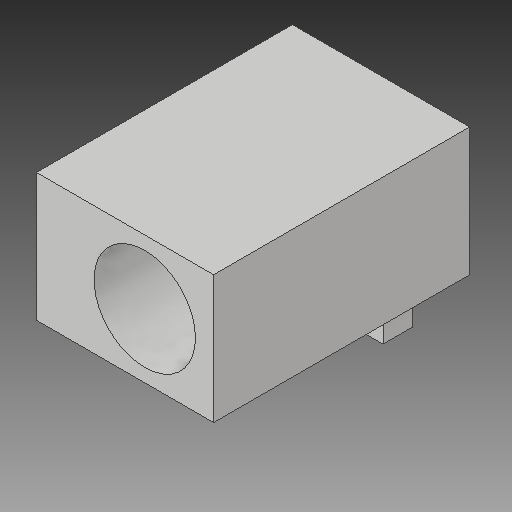
# Autodesk Inventor part: Circuit_DCjack_HEC3110-01-010
Saved by Autodesk Inventor 2018.3 (Build 223284000, 284)
## iProperties
Created: 2018-02-15
Part Number: Circuit_DCjack_HEC3110-01-010
Material: 一般
Document SubType Name: Modeling
Designer: sktom
Density: 1 g/cm^3
Appearance: 既定
Author: sktom
Title: Circuit_DCjack_HEC3110-01-010
Autodesk Inventor part; units mm, degrees
ref_plane "YZ Plane" through (0, 0, 0) normal (1, 0, 0) x (0, 1, 0)
ref_plane "XZ Plane" through (0, 0, 0) normal (0, 1, 0) x (-1, 0, 0)
ref_plane "XY Plane" through (0, 0, 0) normal (0, 0, 1) x (1, 0, 0)
sketch "スケッチ1" plane through (0, 0, 0) normal (0, 0, 1) x (1, 0, 0)
  line L0 (-5.5, 3.25) -> (3.5, 3.25)
  line L1 (3.5, 3.25) -> (3.5, -3.25)
  line L2 (3.5, -3.25) -> (-5.5, -3.25)
  line L3 (-5.5, -3.25) -> (-5.5, 3.25)
  line L4 (-5.5, 3.25) -> (3.5, -3.25) construction
  line L5 (3.5, 3.25) -> (-5.5, -3.25) construction
  circle A0 centre (0, 0) radius 2.575
  point P0 (-1, 0)
  point P1 (-1, 0)
  dimension "d0" = 5.15
  dimension "d1" = 9
  dimension "d2" = 3.5
  dimension "d3" = 6.5
  constraints: 12 end point, 3 midpoint, 2 parallel, 1 centre point, 1 coincident, 1 horizontal, 1 horizontal alignment, 1 perpendicular
  measures "d0" diameter of A0
  measures "d1" distance of L0.start L0.end
  measures "d2" distance from line of point (0, 0) L1
  measures "d3" distance of L0.end L1.end
extrude "押し出し1" add sketch "スケッチ1" against normal blind 13
sketch "スケッチ2" plane through (-5.5, -3.25, 0) normal (0, -1, 0) x (1, 0, 0)
  circle A0 centre (7, -5) radius 0.75
  circle A1 centre (2, -5) radius 0.75
  line L0 (9, 0) -> (0, 0) projected
  point P0 (5.5, 0)
  dimension "d6" = 1.5
  dimension "d7" = 5
  dimension "d8" = 1.5
  dimension "d9" = 3.5
  constraints: 2 centre point, 1 equal radius, 1 horizontal alignment
  measures "d6" diameter of A1
  measures "d7" distance from line of L0 A0.centre
  measures "d8" horizontal distance of point (5.5, 0) A0.centre
  measures "d9" horizontal distance of point (5.5, 0) A1.centre
extrude "押し出し2" add sketch "スケッチ2" along normal blind 1
sketch "スケッチ3" plane through (-5.5, -3.25, 0) normal (0, -1, 0) x (1, 0, 0)
  line L0 (4.15, -10.75) -> (6.85, -10.75)
  line L1 (6.85, -10.75) -> (6.85, -12.25)
  line L2 (6.85, -12.25) -> (4.15, -12.25)
  line L3 (4.15, -12.25) -> (4.15, -10.75)
  line L4 (4.15, -10.75) -> (6.85, -12.25) construction
  line L5 (6.85, -10.75) -> (4.15, -12.25) construction
  circle A0 centre (7, -5) radius 0.75 projected
  line L6 (1.7, -11.3) -> (2.5, -11.3)
  line L7 (2.5, -11.3) -> (2.5, -13.3)
  line L8 (2.5, -13.3) -> (1.7, -13.3)
  line L9 (1.7, -13.3) -> (1.7, -11.3)
  line L10 (1.7, -11.3) -> (2.5, -13.3) construction
  line L11 (2.5, -11.3) -> (1.7, -13.3) construction
  line L12 (0.2, -7.8) -> (1, -7.8)
  line L13 (1, -7.8) -> (1, -9.8)
  line L14 (1, -9.8) -> (0.2, -9.8)
  line L15 (0.2, -9.8) -> (0.2, -7.8)
  line L16 (0.2, -7.8) -> (1, -9.8) construction
  line L17 (1, -7.8) -> (0.2, -9.8) construction
  circle A1 centre (2, -5) radius 0.75 projected
  point P0 (5.5, 0)
  point P1 (5.5, -11.5)
  point P2 (5.5, -11.5)
  point P3 (2.1, -12.3)
  point P4 (0.6, -8.8)
  dimension "d12" = 1.5
  dimension "d13" = 2.7
  dimension "d15" = 6.5
  dimension "d16" = 0.8
  dimension "d17" = 2
  dimension "d18" = 4.9
  dimension "d19" = 3.8
  dimension "d20" = 3.4
  dimension "d21" = 7.3
  constraints: 36 end point, 8 parallel, 7 midpoint, 3 horizontal, 3 perpendicular, 1 vertical alignment
  measures "d12" distance of L0.end L1.end
  measures "d13" distance of L0.start L0.end
  measures "d15" vertical distance of A0.centre point (5.5, -11.5)
  measures "d16" distance of L12.start L12.end
  measures "d17" distance of L14.end L12.start
  measures "d18" horizontal distance of point (5.5, 0) point (0.6, -8.8)
  measures "d19" vertical distance of A1.centre point (0.6, -8.8)
  measures "d20" horizontal distance of point (5.5, 0) point (2.1, -12.3)
  measures "d21" vertical distance of point (2.1, -12.3) A1.centre
extrude "押し出し3" add sketch "スケッチ3" along normal blind 3 contours L0 L1 L2 L3 | L6 L7 L8 L9 | L12 L13 L14 L15
sketch "スケッチ4" plane through (0, 0, -13) normal (0, 0, -1) x (-1, 0, 0)
  line L0 (-3.5, 3.25) -> (-3.5, -3.25) projected
  line L1 (5.5, -3.25) -> (5.5, 3.25) projected
  line L2 (-3.5, 3.25) -> (5.5, 3.25)
  line L3 (5.5, 3.25) -> (5.5, -3.25)
  line L4 (5.5, -3.25) -> (-3.5, -3.25)
  line L5 (-3.5, -3.25) -> (-3.5, 3.25)
  point P0 (0, 0)
  constraints: 8 end point, 2 parallel, 1 horizontal, 1 perpendicular
extrude "押し出し4" add sketch "スケッチ4" against normal blind 3
